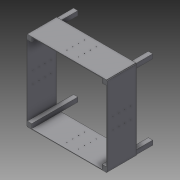
# Autodesk Inventor part: Monitor Mount
Saved by Autodesk Inventor 2013 (Build 170138000, 138)
## iProperties
Created: 2013-03-16
Part Number: Monitor Mount
Material: Generic
Document SubType Name: Modeling
Designer: tyler.camp
Density: 1 g/cm^3
Author: tyler.camp
Autodesk Inventor part; units mm, degrees
ref_plane "YZ Plane" through (0, 0, 0) normal (1, 0, 0) x (0, 1, 0)
ref_plane "XZ Plane" through (0, 0, 0) normal (0, 1, 0) x (-1, 0, 0)
ref_plane "XY Plane" through (0, 0, 0) normal (0, 0, 1) x (1, 0, 0)
sketch "Sketch1" plane through (0, 0, 0) normal (0, 0, 1) x (1, 0, 0)
  line L0 (-342.9, 342.9) -> (-304.8, 342.9)
  line L1 (-304.8, 342.9) -> (-304.8, 304.8)
  line L2 (-304.8, 304.8) -> (-342.9, 304.8)
  line L3 (-342.9, 304.8) -> (-342.9, 342.9)
  line L4 (304.8, 342.9) -> (342.9, 342.9)
  line L5 (342.9, 342.9) -> (342.9, 304.8)
  line L6 (342.9, 304.8) -> (304.8, 304.8)
  line L7 (304.8, 304.8) -> (304.8, 342.9)
  line L8 (342.9, -342.9) -> (304.8, -342.9)
  line L9 (304.8, -342.9) -> (304.8, -304.8)
  line L10 (304.8, -304.8) -> (342.9, -304.8)
  line L11 (342.9, -304.8) -> (342.9, -342.9)
  line L12 (-342.9, -304.8) -> (-304.8, -304.8)
  line L13 (-304.8, -304.8) -> (-304.8, -342.9)
  line L14 (-304.8, -342.9) -> (-342.9, -342.9)
  line L15 (-342.9, -342.9) -> (-342.9, -304.8)
  point P0 (0, 0)
  dimension "d6" = 38.1
  dimension "d9" = 609.6
  dimension "d11" = 304.8
  dimension "d12" = 609.6
  dimension "d13" = 304.8
  constraints: 32 end point, 8 parallel, 7 equal length, 4 collinear, 4 horizontal, 4 perpendicular, 1 other
  measures "d6" distance of L0.end L1.end
  measures "d9" distance between parallel lines of L7 L1
  measures "d11" distance from line of L1 point (0, 0)
  measures "d12" distance between parallel lines of L6 L10
  measures "d13" distance from line of point (0, 0) L10
extrude "Extrusion1" add sketch "Sketch1" along normal blind 400
sketch "Sketch6" plane through (342.9, -342.9, 0) normal (1, 0, 0) x (0, 0, -1)
  line L0 (0, 0) -> (-400, 0) projected
  line L1 (0, 685.8) -> (0, 647.7) projected
  line L2 (0, 685.8) -> (-400, 685.8) projected
  line L3 (-400, 647.7) -> (-400, 685.8) projected
  line L4 (0, 647.7) -> (-400, 647.7) projected
  line L5 (-400, 0) -> (-146, 0)
  line L6 (-146, 0) -> (-146, 685.8)
  line L7 (-146, 685.8) -> (-400, 685.8)
  line L8 (-400, 685.8) -> (-400, 0)
  point P0 (0, 342.9)
  dimension "d31" = 254
  constraints: 8 end point, 2 parallel, 2 point on line, 1 horizontal, 1 perpendicular
  measures "d31" distance between parallel lines of L8 L6
extrude "Extrusion4" add sketch "Sketch6" along normal blind 5 contours L0 L8 L4 L6 | L4 L3 L2 L6
sketch "Sketch7" plane through (347.9, -342.9, 0) normal (1, 0, 0) x (0, 0, -1)
  line L0 (-400, 685.8) -> (-400, 0) projected
  circle A0 centre (-349.2, 292.1) radius 2.5
  line L1 (-146, 38.1) -> (-146, 0) projected
  line L2 (0, 0) -> (-146, 0) projected
  line L3 (0, 38.1) -> (0, 0) projected
  line L4 (0, 38.1) -> (-146, 38.1) projected
  line L5 (-146, 685.8) -> (-146, 647.7) projected
  line L6 (0, 647.7) -> (-146, 647.7) projected
  line L7 (0, 685.8) -> (0, 647.7) projected
  line L8 (0, 685.8) -> (-146, 685.8) projected
  circle A1 centre (-349.2, 393.7) radius 2.5
  circle A2 centre (-298.4, 292.1031) radius 2.5
  circle A3 centre (-298.4, 393.7031) radius 2.5
  circle A4 centre (-247.6, 292.1) radius 2.5
  circle A5 centre (-247.6, 393.7) radius 2.5
  circle A6 centre (-196.8, 292.1) radius 2.5
  circle A7 centre (-196.8, 393.7) radius 2.5
  point P0 (0, 342.9)
  point P1 (-400, 38.1)
  dimension "d38" = 5
  dimension "d40" = 50.8
  dimension "d41" = 609.6
  dimension "d42" = 254
  dimension "d44" = 101.6
  dimension "d48" = 101.6
  dimension "d49" = 101.6
  dimension "d51" = 101.6
  dimension "d63" = 50.8
  dimension "d64" = 50.8
  dimension "d65" = 50.8
  dimension "d66" = 50.8
  dimension "d67" = 50.8
  dimension "d68" = 50.8
  dimension "d69" = 50.8
  constraints: 8 centre point, 4 equal radius
  measures "d38" diameter of A0
  measures "d40" distance from line of L0 A0.centre
  measures "d41" distance between parallel lines of L6 L4
  measures "d42" distance from line of L4 A0.centre
  measures "d44" distance of A1.centre A0.centre
  measures "d48" distance of A3.centre A2.centre
  measures "d49" distance of A5.centre A4.centre
  measures "d51" distance of A7.centre A6.centre
  measures "d63" distance of A0.centre A2.centre
  measures "d64" distance of A1.centre A3.centre
  measures "d65" distance of A2.centre A4.centre
  measures "d66" distance of A3.centre A5.centre
  measures "d67" distance from line of L0 A1.centre
  measures "d68" distance of A6.centre A4.centre
  measures "d69" distance of A5.centre A7.centre
extrude "Extrusion5" cut sketch "Sketch7" against normal up to next contours A0 | A1 | A2 | A3 | A4 | A5 | A6 | A7
pattern_circular "Circular Pattern2" count 4 over 360 about axis through (0, 0, -10) along (0, 0, 1) of "Extrusion4", "Extrusion5"
equation "\"d11\" = 0.5 * d9"
equation "\"d12\" = d9"
equation "\"d13\" = 0.5 * d12"
equation "\"d48\" = d44"
equation "\"d49\" = d44"
equation "\"d51\" = d44"
equation "\"d65\" = d63"
equation "\"d66\" = d64"
equation "\"d67\" = d40"
equation "\"d68\" = d65"
body "Solid1"
